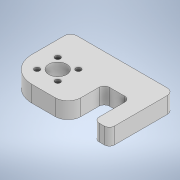
# Autodesk Inventor part: platform hook
Saved by Autodesk Inventor 2020 (Build 240168000, 168)
## iProperties
Created: 2019-12-20
Part Number: platform hook
Material: Generic
Document SubType Name: Modeling
Designer: xj82b
Density: 1 g/cm^3
Appearance: Default
Author: xj82b
Autodesk Inventor part; units mm, degrees
ref_plane "YZ Plane" through (0, 0, 0) normal (1, 0, 0) x (0, 1, 0)
ref_plane "XZ Plane" through (0, 0, 0) normal (0, 1, 0) x (-1, 0, 0)
ref_plane "XY Plane" through (0, 0, 0) normal (0, 0, 1) x (1, 0, 0)
sketch "Sketch1" plane through (0, 0, 0) normal (0, 1, 0) x (-1, 0, 0)
  line L0 (-84, -3) -> (-84, -35)
  line L1 (-80, -39) -> (-24, -39)
  line L2 (-52, -9) -> (-52, -23)
  line L3 (-56, -27) -> (-68, -27)
  line L4 (-72, -23) -> (-72, -3)
  line L5 (-24, 1) -> (-42, 1)
  line L6 (-76, 1) -> (-80, 1)
  arc A0 (-80, 1) -> (-84, -3) centre (-80, -3) ccw
  arc A1 (-72, -3) -> (-76, 1) centre (-76, -3) ccw
  arc A2 (-84, -35) -> (-80, -39) centre (-80, -35) ccw
  arc A3 (-72, -23) -> (-68, -27) centre (-68, -23) ccw
  arc A4 (-56, -27) -> (-52, -23) centre (-56, -23) ccw
  arc A5 (-24, -39) -> (-24, 1) centre (-24, -19) ccw
  arc A6 (-42, 1) -> (-52, -9) centre (-42, -9) ccw
  line L7 (-4, -19) -> (-4, -49)
  line L8 (-4, -49) -> (-84, -49)
  line L9 (-84, -49) -> (-84, -35)
  point P0 (-84, -39)
  point P1 (-52, -27)
  point P2 (-52, 1)
  point P3 (-72, -27)
  dimension "d2" = 20
  dimension "d4" = 12
  dimension "d6" = 40
  dimension "d9" = 40
  dimension "d24" = 4
  dimension "d25" = 10
  dimension "d26" = 28
  dimension "d27" = 12
  dimension "d32" = 30
  constraints: 20 end point, 15 point on circle, 14 tangent, 8 point on line, 7 centre point, 4 equal radius, 4 perpendicular, 3 parallel, 2 horizontal, 2 vertical alignment, 1 collinear, 1 vertical
  measures "d2" distance of point (-52, -27) point (-72, -27)
  measures "d4" distance between parallel lines of L0 L4
  measures "d6" distance between parallel lines of L1 L6
  measures "d9" diameter of A5
  measures "d24" radius of A0
  measures "d25" radius of A6
  measures "d26" distance from line of A5.centre L2
  measures "d27" distance between parallel lines of L1 L3
  measures "d32" distance of L7.start L7.end
extrude "Extrusion1" add sketch "Sketch1" along normal blind 12.7
sketch "Sketch2" plane through (0, 12.7, 0) normal (0, 1, 0) x (1, 0, 0)
  circle A0 centre (24, 19) radius 7
  arc A1 (4, 19) -> (24, -1) centre (24, 19) ccw projected
  circle A2 centre (32, 27) radius 2.05
  circle A3 centre (16, 27) radius 2.05
  circle A4 centre (16, 11) radius 2.05
  circle A5 centre (32, 11) radius 2.05
  point P0 (0, 0)
  point P1 (24, 39)
  dimension "d13" = 14
  dimension "d14" = 4.1
  dimension "d15" = 4.1
  dimension "d16" = 4.1
  dimension "d17" = 4.1
  dimension "d18" = 16
  dimension "d19" = 16
  dimension "d20" = 8
  dimension "d21" = 8
  constraints: 5 centre point, 2 horizontal alignment, 2 vertical alignment, 1 concentric
  measures "d13" diameter of A0
  measures "d14" diameter of A2
  measures "d15" diameter of A3
  measures "d16" diameter of A4
  measures "d17" diameter of A5
  measures "d18" distance of A5.centre A2.centre
  measures "d19" distance of A4.centre A5.centre
  measures "d20" horizontal distance of A0.centre A2.centre
  measures "d21" horizontal distance of A0.centre A5.centre
extrude "Extrusion2" cut sketch "Sketch2" against normal through all
fillet "Fillet1" radius 5 2 edges at (84, 6.35, -49) (4, 6.35, -49)
body "Solid1"
